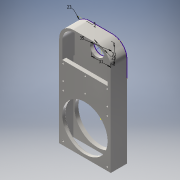
# Autodesk Inventor part: Cup_Dispenser_Hull
Saved by Autodesk Inventor 2016 (Build 200138000, 138)
## iProperties
Created: 2015-07-04
Part Number: Cup_Dispenser_Hull
Material: Generic
Document SubType Name: Modeling
Designer: marku
Density: 1 g/cm^3
Appearance: Titanium
Author: marku
Autodesk Inventor part; units mm, degrees
ref_plane "YZ Plane" through (0, 0, 0) normal (1, 0, 0) x (0, 1, 0)
ref_plane "XZ Plane" through (0, 0, 0) normal (0, 1, 0) x (-1, 0, 0)
ref_plane "XY Plane" through (0, 0, 0) normal (0, 0, 1) x (1, 0, 0)
derived "Cup_Dispenser_Slider.ipt"
sketch "Sketch13" plane through (0, 0, 0) normal (0, 1, 0) x (-1, 0, 0)
  circle A0 centre (0, 0) radius 35 construction
  circle A1 centre (0, 0) radius 31.375 construction
  line L0 (0, 60.7625) -> (0, -56.1294) construction
  line L1 (45.182, 0) -> (-48.0239, 0) construction
  circle A2 centre (0, 35) radius 35 construction
  circle A3 centre (0, 35) radius 31.375 construction
  line L2 (31.375, 35) -> (31.375, 19.4884)
  line L3 (35, 19.4884) -> (35, 70)
  line L4 (35, 70) -> (0, 70)
  line L5 (31.375, 19.4884) -> (35, 19.4884)
  arc A4 (31.375, 35) -> (0, 66.375) centre (0, 35) ccw
  line L6 (0, 70) -> (0, 66.375) construction
  line L7 (0, 31.375) -> (0, 3.625) construction
  line L8 (0, 17.5) -> (45.182, 17.5) construction
  line L9 (-35, 19.4884) -> (-35, 70)
  line L10 (-35, 70) -> (0, 70)
  line L11 (-31.375, 19.4884) -> (-35, 19.4884)
  line L12 (-31.375, 35) -> (-31.375, 19.4884)
  arc A5 (0, 66.375) -> (-31.375, 35) centre (0, 35) ccw
  line L13 (35, 15.5116) -> (35, -35)
  line L14 (31.375, 15.5116) -> (35, 15.5116)
  line L15 (31.375, 0) -> (31.375, 15.5116)
  arc A6 (0, -31.375) -> (31.375, 0) centre (0, 0) ccw
  line L16 (35, -35) -> (0, -35)
  line L17 (-35, -35) -> (0, -35)
  arc A7 (-31.375, 0) -> (0, -31.375) centre (0, 0) ccw
  line L18 (-35, 15.5116) -> (-35, -35)
  line L19 (-31.375, 15.5116) -> (-35, 15.5116)
  line L20 (-31.375, 0) -> (-31.375, 15.5116)
  line L21 (35, 70) -> (35, -35)
  line L22 (-35, -35) -> (-35, 70)
  line L23 (-38, 73) -> (38, 73)
  line L24 (38, 73) -> (38, -38)
  line L25 (38, -38) -> (-38, -38)
  line L26 (-38, -38) -> (-38, 73)
  line L27 (-38, 73) -> (38, -38) construction
  line L28 (38, 73) -> (-38, -38) construction
sketch "Sketch2" plane through (0, 0, 0) normal (0, 1, 0) x (-1, 0, 0)
  line L0 (-41, 76) -> (41, 76)
  line L1 (41, 76) -> (41, -41)
  line L2 (41, -41) -> (-41, -41)
  line L3 (-41, -41) -> (-41, 76)
  line L4 (-41, 76) -> (41, -41) construction
  line L5 (41, 76) -> (-41, -41) construction
  line L6 (38, -38) -> (38, 73)
  line L7 (38, 73) -> (-38, 73)
  line L8 (-38, 73) -> (-38, -38)
  line L9 (-38, -38) -> (38, -38)
  line L10 (-35, 35) -> (35, 35) construction
  line L11 (35, 35) -> (35, -35) construction
  line L12 (35, -35) -> (-35, -35) construction
  line L13 (-35, -35) -> (-35, 35) construction
  line L14 (-35, 35) -> (35, -35) construction
  line L15 (35, 35) -> (-35, -35) construction
  circle A0 centre (0, 0) radius 36
  point P0 (0, 17.5)
  dimension "d1" = 82
  dimension "d2" = 117
  dimension "d3" = 3
  dimension "d4" = 70
  dimension "d5" = 70
  dimension "d8" = 72
  constraints: 32 end point, 6 parallel, 5 coincident, 4 midpoint, 3 perpendicular, 2 horizontal, 1 centre point, 3 other
  measures "d1" distance of L1.end L2.end
  measures "d2" distance of L0.end L1.end
  measures "d3" distance between parallel lines of L1 L6
  measures "d4" distance of L11.end L12.end
  measures "d5" distance of L10.end L11.end
  measures "d8" diameter of A0
extrude "Extrusion1" add sketch "Sketch2" against normal blind 6 contours L0 L1 L2 L3 | L9 L8 L7 L6
extrude "Extrusion2" add sketch "Sketch2" against normal blind 19.5 contours L0 L1 L2 L3
sketch "Sketch3" plane through (0, -19.5, 0) normal (0, -1, 0) x (1, 0, 0)
  line L0 (41, -41) -> (41, 76) projected
  line L1 (41, 76) -> (-41, 76) projected
  line L2 (-41, 76) -> (-41, -41) projected
  line L3 (-41, -41) -> (41, -41) projected
  circle A0 centre (0, 0) radius 36 projected
extrude "Extrusion3" add sketch "Sketch3" along normal blind 3
hole "Hole1" at (0, 0, 17.5) at (-35, 0, 35) at (-35, 0, -35) at (35, 0, -35) at (35, 0, 35) direction (0, -1, 0) diameter 3 depth 4 tip angle 118
chamfer "Chamfer1" distance 2 angle 45 2 edges at (-38, -12.75, 73) (38, -12.75, 73)
sketch "Sketch4" plane through (41, 0, -41) normal (0, 0, -1) x (-1, 0, 0)
  line L0 (79, -6) -> (3, -6) projected
  line L1 (79, -6) -> (79, -19.5) projected
  line L2 (3, -19.5) -> (79, -19.5) projected
  line L3 (3, -6) -> (3, -19.5) projected
  point P0 (41, 0)
extrude "Extrusion4" cut sketch "Sketch4" against normal blind 3
sketch "Sketch11" plane through (-39, -22.5, 76) normal (0, 0, 1) x (1, 0, 0)
  line L0 (75, 16.5) -> (3, 16.5) projected
  line L1 (3, 16.5) -> (3, 3) projected
  line L2 (3, 3) -> (75, 3) projected
  line L3 (75, 3) -> (75, 16.5) projected
  point P0 (39, 22.5)
extrude "Extrusion8" cut sketch "Sketch11" against normal blind 3
sketch "Sketch15" plane through (0, 0, 0) normal (0, 1, 0) x (1, 0, 0)
  line L0 (-15.5, -115) -> (15.5, -115) construction
  line L1 (15.5, -115) -> (15.5, -84) construction
  line L2 (15.5, -84) -> (-15.5, -84) construction
  line L3 (-15.5, -84) -> (-15.5, -115) construction
  line L4 (-15.5, -115) -> (15.5, -84) construction
  line L5 (15.5, -115) -> (-15.5, -84) construction
  line L6 (41, -76) -> (-41, -76) projected
  arc A0 (-36, -103) -> (-16, -123) centre (-16, -103) ccw construction
  arc A1 (16, -123) -> (36, -103) centre (16, -103) ccw construction
  circle A2 centre (0, -99.5) radius 17.5 construction
  line L7 (0, -123) -> (0, -57.6471) construction
  circle A3 centre (0, -99.5) radius 11.5
  line L8 (36, -123) -> (-36, -123) construction
  line L9 (-41, -76) -> (-41, -103)
  line L10 (-18, -126) -> (18, -126)
  line L11 (41, -103) -> (41, -76)
  arc A4 (-41, -103) -> (-18, -126) centre (-18, -103) ccw
  arc A5 (18, -126) -> (41, -103) centre (18, -103) ccw
  point P0 (0, 0)
  point P1 (0, -117)
  dimension "d66" = 35
  dimension "d60" = 31
  dimension "d61" = 31
  dimension "d67" = 23
  dimension "d68" = 3
  dimension "d69" = 23
  constraints: 18 end point, 5 coincident, 4 point on circle, 4 tangent, 3 centre point, 3 perpendicular, 2 parallel, 1 equal radius, 1 horizontal, 1 midpoint, 1 point on line, 1 vertical, 1 vertical alignment, 2 other
  measures "d60" distance of L2.end L1.end
  measures "d61" distance of L1.end L0.end
  measures "d67" diameter of A3
  measures "d68" distance between parallel lines of L10 L8
  measures "d69" radius of A4
extrude "Extrusion9" add sketch "Sketch15" against normal blind 6
sketch "Sketch16" plane through (0, 0, 0) normal (0, 1, 0) x (1, 0, 0)
  line L0 (-36, -73) -> (-36, -103) projected
  arc A0 (-36, -103) -> (-16, -123) centre (-16, -103) ccw projected
  line L1 (16, -123) -> (-16, -123) projected
  arc A1 (16, -123) -> (36, -103) centre (16, -103) ccw projected
  line L2 (36, -103) -> (36, -73) projected
  arc A2 (-41, -103) -> (-18, -126) centre (-18, -103) ccw projected
  line L3 (-18, -126) -> (18, -126) projected
  arc A3 (18, -126) -> (41, -103) centre (18, -103) ccw projected
  line L4 (-41, -103) -> (-41, -73)
  line L5 (-41, 41) -> (-41, -103) projected
  line L6 (-36, -73) -> (-41, -73)
  line L7 (41, -103) -> (41, -73)
  line L8 (41, 41) -> (41, -103) projected
  line L9 (36, -73) -> (41, -73)
  point P0 (0, 0)
  constraints: 8 end point, 2 perpendicular, 2 point on line
extrude "Extrusion10" add sketch "Sketch16" against normal up to surface (22.5 mm away)
hole "Hole3" at (-15.5, 0, 84) at (15.5, 0, 84) at (-15.5, 0, 115) at (15.5, 0, 115) direction (0, -1, 0) diameter 3 depth 4 tip angle 118
sketch "Sketch17" plane through (0, -22.5, 0) normal (0, -1, 0) x (1, 0, 0)
  line L0 (-41, -41) -> (-41, 103) projected
  line L1 (-41, -41) -> (41, -41) projected
  line L2 (41, -41) -> (41, 103) projected
  arc A0 (41, 103) -> (18, 126) centre (18, 103) ccw projected
  line L3 (-18, 126) -> (18, 126) projected
  arc A1 (-18, 126) -> (-41, 103) centre (-18, 103) ccw projected
  circle A2 centre (0, 0) radius 36 projected
  line L4 (-36, 103) -> (-36, 76) projected
  arc A3 (-16, 123) -> (-36, 103) centre (-16, 103) ccw projected
  line L5 (16, 123) -> (-16, 123) projected
  arc A4 (36, 103) -> (16, 123) centre (16, 103) ccw projected
  line L6 (36, 76) -> (36, 103) projected
  line L7 (36, 76) -> (-36, 76) projected
extrude "Extrusion11" add sketch "Sketch17" along normal blind 3
sketch "Sketch18" plane through (0, 0, 0) normal (0, 1, 0) x (1, 0, 0)
  line L0 (35, -72) -> (-35, -72)
  line L1 (-35, -72) -> (-35, -48)
  line L2 (-35, -48) -> (35, -48)
  line L3 (35, -48) -> (35, -72)
  line L4 (35, -72) -> (-35, -48) construction
  line L5 (-35, -72) -> (35, -48) construction
  line L6 (-41, 41) -> (-41, -103) projected
  line L7 (0, -123) -> (0, -57.6471) construction
  point P0 (0, 0)
  point P1 (0, -60)
  point P2 (0, -72)
  point P3 (0, -48)
  dimension "d81" = 6
  dimension "d96" = 24
  dimension "d97" = 48
  constraints: 12 end point, 4 coincident, 4 midpoint, 2 parallel, 1 horizontal, 1 perpendicular, 1 point on line, 1 other
  measures "d81" distance between parallel lines of L6 L1
  measures "d96" distance between parallel lines of L2 L0
  measures "d97" distance from line of point (0, 0) L2
hole "Hole4" at (-35, 0, 72) at (-35, 0, 48) at (35, 0, 48) at (35, 0, 72) at (0, 0, 72) at (0, 0, 48) direction (0, -1, 0) diameter 3 depth 4 tip angle 118
sketch "Sketch19" plane through (0, -25.5, 0) normal (0, -1, 0) x (1, 0, 0)
  circle A0 centre (35, 72) radius 1.5 projected
  circle A1 centre (0, 72) radius 1.5 projected
  circle A2 centre (-35, 72) radius 1.5 projected
  circle A3 centre (-35, 48) radius 1.5 projected
  circle A4 centre (0, 48) radius 1.5 projected
  circle A5 centre (35, 48) radius 1.5 projected
  circle A6 centre (35, 35) radius 1.5 projected
  circle A7 centre (-35, 35) radius 1.5 projected
  circle A8 centre (-35, -35) radius 1.5 projected
  circle A9 centre (-35, -35) radius 1.5 projected
  circle A10 centre (35, -35) radius 1.5 projected
  point P0 (0, 0)
hole "Hole5" at (35, -25.5, 72) at (35, -25.5, 48) at (35, -25.5, 35) at (35, -25.5, -35) at (-35, -25.5, -35) at (-35, -25.5, 35) at (-35, -25.5, 48) at (-35, -25.5, 72) at (0, -25.5, 72) at (0, -25.5, 48) direction (0, 1, 0) diameter 3 depth 4 tip angle 118
fillet "Fillet2" radius 2 1 edges at (-36, -19.5, 0)
sketch "Sketch21" plane through (0, 0, 0) normal (0, 1, 0) x (1, 0, 0)
  circle A0 centre (0, -72) radius 1.5 projected
  circle A1 centre (35, -48) radius 1.5 projected
  circle A2 centre (-35, -72) radius 1.5 projected
  circle A3 centre (-35, -48) radius 1.5 projected
  circle A4 centre (35, -72) radius 1.5 projected
  circle A5 centre (0, -48) radius 1.5 projected
  circle A6 centre (-15.5, -115) radius 1.5 projected
  circle A7 centre (-15.5, -84) radius 1.5 projected
  circle A8 centre (15.5, -84) radius 1.5 projected
  circle A9 centre (15.5, -115) radius 1.5 projected
  circle A10 centre (0, 0) radius 36 projected
  line L0 (-41, 41) -> (-41, -103) projected
  arc A11 (-41, -103) -> (-18, -126) centre (-18, -103) ccw projected
  line L1 (-18, -126) -> (18, -126) projected
  arc A12 (18, -126) -> (41, -103) centre (18, -103) ccw projected
  line L2 (41, 41) -> (41, -103) projected
  line L3 (-41, 41) -> (41, 41) projected
  circle A13 centre (35, -35) radius 1.5 projected
  circle A14 centre (-35, 35) radius 1.5 projected
  circle A15 centre (-35, -35) radius 1.5 projected
  circle A16 centre (35, 35) radius 1.5 projected
  circle A17 centre (0, -99.5) radius 11.5 projected
  line L4 (0, -136.0201) -> (0, 47.5544) construction
  circle A18 centre (-18, -60.7956) radius 14.3193
  circle A19 centre (-25.2211, -97.6989) radius 9.0279
  circle A20 centre (18, -60.7956) radius 14.3193
  circle A21 centre (25.2211, -97.6989) radius 9.0279
  constraints: 4 centre point, 2 end point, 2 symmetric about line, 1 point on line, 1 vertical, 2 other
extrude "Extrusion12" cut sketch "Sketch21" against normal blind 2 contours A18 | A19 | A20 | A21
body "Solid1"
